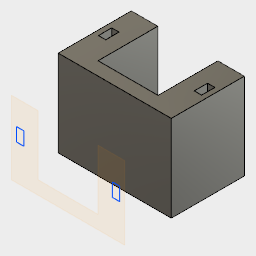
Motor casing v5 (Autodesk Fusion 360 design; units mm, degrees)
Autodesk Fusion 360 part; units mm, degrees
sketch "Sketch1" plane through (0, 0, 0) normal (0, 1, 0) x (1, 0, 0)
  line L0 (-40, 20) -> (45, 20)
  line L1 (45, 20) -> (45, -35)
  line L2 (45, -35) -> (-40, -35)
  line L3 (-40, -35) -> (-40, 20)
  dimension "d1" = 85
  dimension "d2" = 55
  measures "d1" distance of L0.start L0.end
  measures "d2" distance of L0.start L2.end
extrude "Extrude1" add sketch "Sketch1" along normal blind 10
sketch "Sketch2" plane through (0, 10, 0) normal (0, 1, 0) x (-1, 0, 0)
  line L0 (40, 35) -> (-45, 35)
  line L1 (-45, 35) -> (-45, -20)
  line L2 (-45, -20) -> (40, -20)
  line L3 (40, -20) -> (40, 35)
  line L4 (-45, -20) -> (-25, -20)
  line L5 (-25, -20) -> (-25, 35)
  line L6 (-25, 35) -> (-45, 35)
  line L7 (-45, 35) -> (-45, -20)
  dimension "d5" = 20
  measures "d5" distance of L1.end L4.end
extrude "Extrude2" add sketch "Sketch2" along normal blind 45 contours L0 L1 L2 L4 L5 L6 L7
sketch "Sketch3" plane through (0, 10, 0) normal (0, 1, 0) x (-1, 0, 0)
  line L0 (-25, 35) -> (-25, -20)
  line L1 (-25, -20) -> (40, -20)
  line L2 (40, -20) -> (40, 35)
  line L3 (40, 35) -> (-25, 35)
  line L4 (40, -20) -> (20, -20)
  line L5 (20, -20) -> (20, 35)
  line L6 (20, 35) -> (40, 35)
  line L7 (40, 35) -> (40, -20)
  dimension "d8" = 20
  measures "d8" distance of L1.end L4.end
extrude "Extrude3" add sketch "Sketch3" along normal blind 45 contours L1 L2 L3 L4 L5 L6 L7
sketch "Sketch4" plane through (0, 0, 0) normal (0, 1, 0) x (1, 0, 0)
  line L0 (-40, 20) -> (45, 20)
  line L1 (45, 20) -> (45, 30)
  line L2 (45, 30) -> (-40, 30)
  line L3 (-40, 30) -> (-40, 20)
  point P0 (-40, 20)
  dimension "d11" = 10
  measures "d11" distance of P0 L2.end
extrude "Extrude4" add sketch "Sketch4" along normal blind 55
sketch "Sketch5" plane through (0, 0, 35) normal (0, 0, 1) x (1, 0, 0)
  line L0 (-40, 0) -> (45, 0)
  line L1 (45, 0) -> (45, 55)
  line L2 (45, 55) -> (25, 55)
  line L3 (25, 55) -> (25, 10)
  line L4 (25, 10) -> (-20, 10)
  line L5 (-20, 10) -> (-20, 55)
  line L6 (-20, 55) -> (-40, 55)
  line L7 (-40, 55) -> (-40, 0)
  line L8 (-36.25, 36.5) -> (-30.75, 36.5)
  line L9 (-30.75, 36.5) -> (-30.75, 26.5)
  line L10 (-30.75, 26.5) -> (-36.25, 26.5)
  line L11 (-36.25, 26.5) -> (-36.25, 36.5)
  line L12 (35.75, 36.5) -> (41.25, 36.5)
  line L13 (41.25, 36.5) -> (41.25, 26.5)
  line L14 (41.25, 26.5) -> (35.75, 26.5)
  line L15 (35.75, 26.5) -> (35.75, 36.5)
  dimension "d14" = 5.5
  dimension "d15" = 10
  dimension "d16" = 5.5
  dimension "d17" = 10
  measures "d14" distance of L8.start L8.end
  measures "d15" distance of L8.start L10.end
  measures "d16" distance of L12.start L12.end
  measures "d17" distance of L14.end L12.start
extrude "Extrude5" cut sketch "Sketch5" against normal blind 10.5 contours L8 L9 L10 L11
extrude "Extrude6" cut sketch "Sketch5" against normal blind 10.5 contours L12 L13 L14 L15
move_body "Move1" bodies 1 to x (1, 0, 0) y (0, 0, -1) z (0, 1, 0) at (0, 0, 0)
move_body "Move2" bodies 1 to x (1, 0, 0) y (0, 1, 0) z (0, 0, 1) at (0, 30, 0)
